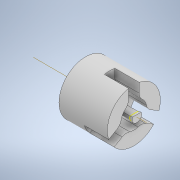
# Autodesk Inventor part: front wheel mount
Saved by Autodesk Inventor 2022.6 (Build 266554000, 554)
## iProperties
Created: 2024-10-28
Part Number: front wheel mount
Material: Generic
Document SubType Name: Modeling
Designer: Zhong
Density: 1 g/cm^3
Appearance: Default
Author: Zhong
Autodesk Inventor part; units mm, degrees
ref_plane "YZ Plane" through (0, 0, 0) normal (1, 0, 0) x (0, 1, 0)
ref_plane "XZ Plane" through (0, 0, 0) normal (0, 1, 0) x (-1, 0, 0)
sketch "Sketch1" plane through (0, 0, 0) normal (1, 0, 0) x (0, 1, 0)
  circle A0 centre (0, 0) radius 1.4
  line L0 (0.5, 1.30767) -> (0.5, -1.30767)
  dimension "d1" = 2.8
  dimension "d2" = 0.5
  constraints: 2 end point, 2 point on circle, 1 centre point, 1 coincident, 1 vertical
  measures "d1" diameter of A0
  measures "d2" distance from line of point (0, 0) L0
extrude "Extrusion1" add sketch "Sketch1" along normal blind 8 contours L0 A0 picked at (-0.62029, 0.295862)
sketch "Sketch2" plane through (0, 0, 0) normal (-1, 0, 0) x (0, 0, 1)
  circle A0 centre (0, 0) radius 8.75
  arc A1 (-1.30767, 0.5) -> (1.30767, 0.5) centre (0, 0) ccw
  dimension "d5" = 17.5
  constraints: 1 centre point, 1 coincident
  measures "d5" diameter of A0
extrude "Extrusion2" add sketch "Sketch2" along normal blind 8
sketch "Sketch3" plane through (0, 0, 0) normal (1, 0, 0) x (0, 1, 0)
  circle A0 centre (0, 0) radius 4.25
  line L0 (4, 1.75) -> (8.573214, 1.75)
  line L1 (4, -1.75) -> (8.573214, -1.75)
  line L2 (-10.5, 0) -> (10.5, 0)
  circle A1 centre (0, 0) radius 8.75
  line L3 (0.5, -1.30767) -> (0.5, 1.30767)
  arc A2 (0.5, 1.30767) -> (0.5, -1.30767) centre (0, 0) ccw
  arc A3 (3.820225, 1.86236) -> (4, 1.75) centre (4, 1.95) ccw
  arc A4 (4, -1.75) -> (3.820225, -1.86236) centre (4, -1.95) ccw
  line L4 (-3.515544, 2.589102) -> (-5.802152, 6.549621)
  line L5 (-0.484456, 4.339102) -> (-2.771063, 8.299621)
  arc A5 (-0.484456, 4.339102) -> (-0.297262, 4.239591) centre (-0.31125, 4.439102) ccw
  arc A6 (-3.522963, 2.377232) -> (-3.515544, 2.589102) centre (-3.68875, 2.489102) ccw
  line L6 (-0.484456, -4.339102) -> (-2.771063, -8.299621)
  line L7 (-3.515544, -2.589102) -> (-5.802152, -6.549621)
  arc A7 (-3.515544, -2.589102) -> (-3.522963, -2.377232) centre (-3.68875, -2.489102) ccw
  arc A8 (-0.297262, -4.239591) -> (-0.484456, -4.339102) centre (-0.31125, -4.439102) ccw
  arc A9 (0.5, 1.30767) -> (0.5, -1.30767) centre (0, 0) ccw
  circle A10 centre (0, 0) radius 5
  line L8 (4, 1.75) -> (3.872983, 1.75)
  line L9 (4, -1.75) -> (3.840573, -1.75)
  line L10 (-0.484456, -4.339102) -> (-0.420947, -4.229102)
  line L11 (-3.515544, -2.589102) -> (-3.452036, -2.479102)
  line L12 (-3.515544, 2.589102) -> (-3.452036, 2.479102)
  line L13 (-0.484456, 4.339102) -> (-0.420947, 4.229102)
  point P0 (-3.522963, -2.377232)
  point P1 (-4.25, 0)
  point P2 (-8.75, 0)
  point P3 (-5.802152, -6.549621)
  point P4 (-0.297262, -4.239591)
  point P5 (-2.771063, -8.299621)
  point P6 (8.573214, -1.75)
  point P7 (-0.297262, 4.239591)
  point P8 (-3.522963, 2.377232)
  point P9 (-5.802152, 6.549621)
  point P10 (3.872983, -1.75)
  dimension "d8" = 8.5
  dimension "d9" = 3.5
  dimension "d10" = 4
  dimension "d14" = 360
  dimension "d22" = 10
  constraints: 24 end point, 12 point on circle, 7 centre point, 5 tangent, 4 parallel, 3 horizontal, 2 coincident, 2 point on line, 2 vertical alignment, 51 other
  measures "d9" distance between parallel lines of L0 L1
  measures "d10" horizontal distance of L0.start point (0, 0)
  measures "d22" diameter of A10
extrude "Extrusion3" add sketch "Sketch3" along normal blind 8 contours A0 A3 L8 | L9 A4 A0 | A0 A5 L5 A10 L0 A3 | A4 L1 A10 L6 A8 A0 | A10 L5 A1 L0 | L1 A1 L6 A10 | A0 L13 A5 | A8 L10 A0 | L2 A10 L4 A6 A0 | A0 A7 L7 A10 L2 | A10 L2 A1 L4 | L7 A1 L2 A10 | A6 L12 A0 | A0 L11 A7
sketch "Sketch4" plane through (-8, 0, 0) normal (-1, 0, 0) x (0, 0, 1)
  circle A0 centre (0, 0) radius 6.65
  dimension "d19" = 13.3
  constraints: 1 centre point, 1 coincident
  measures "d19" diameter of A0
extrude "Extrusion4" cut sketch "Sketch4" against normal blind 5.5
fillet "Fillet1" radius 3 6 edges at (4, 3.873, 1.75) (4, -0.4209, 4.2291) (4, 3.873, -1.75) (4, -0.4209, -4.2291) (4, -3.452, -2.4791) (4, -3.452, 2.4791)
sketch "Sketch5" plane through (-2.5, 0, 0) normal (-1, 0, 0) x (0, 0, 1)
  circle A0 centre (0, 0) radius 2.5
  dimension "d24" = 5
  constraints: 1 centre point, 1 coincident
  measures "d24" diameter of A0
extrude "Extrusion5" [suppressed]
sketch "Sketch6" plane through (-22, 0, 0) normal (-1, 0, 0) x (0, 0, 1)
  arc A0 (-1.2, 0.5) -> (1.2, 0.5) centre (0, 0) ccw projected
  circle A1 centre (0, 0) radius 2.5 projected
ref_plane "Work Plane1" through (9, 0, 0) normal (1, 0, 0) x (0, 0, -1)
sketch "Sketch7" plane through (9, 0, 0) normal (1, 0, 0) x (0, 0, -1)
  arc A0 (-1.30767, 0.5) -> (1.30767, 0.5) centre (0, 0) ccw
  line L0 (1.30767, 0.5) -> (-1.30767, 0.5)
  circle A1 centre (0, 0) radius 1.6
  line L1 (-1.438749, 0.7) -> (1.438749, 0.7)
  dimension "d28" = 3.2
  dimension "d30" = 0.5
  dimension "d31" = 0.7
  constraints: 2 end point, 2 point on circle, 1 centre point, 1 coincident, 1 horizontal
  measures "d28" diameter of A1
  measures "d30" distance from line of point (0, 0) L0
  measures "d31" distance from line of point (0, 0) L1
sketch "Sketch8" plane through (8, 0, 0) normal (1, 0, 0) x (0, 0, -1)
  arc A0 (-1.30767, 0.5) -> (1.30767, 0.5) centre (0, 0) ccw
  line L0 (1.30767, 0.5) -> (-1.30767, 0.5)
sketch "Sketch7 outline for Loft1" plane through (9, 0, 0) normal (1, 0, 0) x (0, 0, -1)
  line L0 (1.438749, 0.7) -> (-1.438749, 0.7)
  arc A0 (-1.438749, 0.7) -> (1.438749, 0.7) centre (0, 0) ccw
loft "Loft1" add profiles "Sketch7 outline for Loft1" section 1 edges at (8, -1.4, 0) (8, 0.5, 0)
sketch "Sketch9" plane through (-2.5, 0, 0) normal (-1, 0, 0) x (0, 0, 1)
  circle A0 centre (0, 0) radius 3.15
  dimension "d36" = 6.3
  constraints: 1 centre point, 1 coincident
  measures "d36" diameter of A0
extrude "Extrusion6" cut sketch "Sketch9" against normal blind 0.4
body "Solid1"
